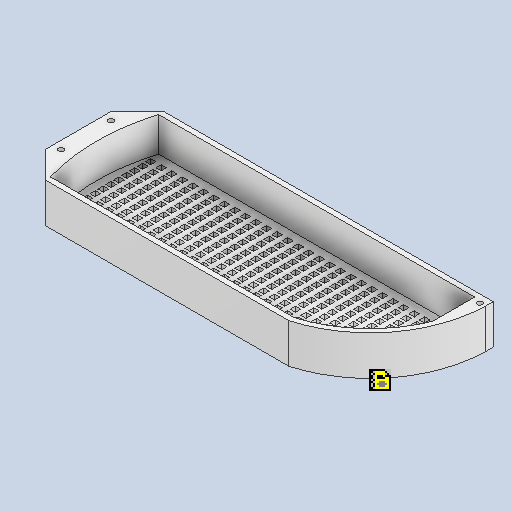
# Autodesk Inventor part: Box
Saved by Autodesk Inventor 2024 (Build 280153000, 153)
## iProperties
Created: 2023-11-02
Part Number: Box
Material: PVC, Unplasticized
Document SubType Name: Modeling
Designer: furqa
Density: 1.29 g/cm^3
Appearance: Smooth - White
Mass: 23.7695 g
Surface Area: 226.35 cm^2
Volume: 18.426 cm^3
Author: furqa
Autodesk Inventor part; units mm, degrees
(part 1 of 2)
ref_plane "YZ Plane" through (0, 0, 0) normal (1, 0, 0) x (0, 1, 0)
ref_plane "XZ Plane" through (0, 0, 0) normal (0, 1, 0) x (-1, 0, 0)
ref_plane "XY Plane" through (0, 0, 0) normal (0, 0, 1) x (1, 0, 0)
sketch "Sketch2" plane through (0, 0, 0) normal (0, 1, 0) x (-1, 0, 0)
  line L0 (0, 0) -> (125, 0)
  line L1 (125, 45) -> (0, 45)
  line L2 (0, 45) -> (0, 0)
  line L3 (125, 45) -> (135, 35)
  line L4 (125, 45) -> (139.1421, 45) construction
  line L5 (125, 0) -> (135, 10)
  line L6 (125, 0) -> (139.1421, 0) construction
  line L7 (135, 35) -> (135, 10)
  dimension "d3" = 45
  dimension "d4" = 45
  constraints: 16 end point, 3 horizontal, 2 equal length, 1 parallel
  measures "d3" angle of L3 L4
  measures "d4" angle of L6 L5
extrude "Extrusion2" add sketch "Sketch2" along normal blind 15
sketch "Sketch3" plane through (-135, 0, 10) normal (-0.7071, 0, -0.7071) x (-0.7071, 0, 0.7071)
  point P0 (-102.5305, 0)
sketch "Sketch4" plane through (0, 15, 0) normal (0, 1, 0) x (1, 0, 0)
  line L0 (-32.5163, -43) -> (-125, -43)
  line L1 (-125, -2) -> (-2, -2)
  line L2 (-2, -2) -> (-2, -4.6897)
  line L3 (0, -45) -> (0, 0) projected
  line L4 (0, 0) -> (-125, 0) projected
  line L5 (-125, -45) -> (0, -45) projected
  line L6 (-135, -10) -> (-135, -35) projected
  arc A0 (-32.5163, -45) -> (0, -1) centre (-44.7799, -1.9222) ccw
  arc A1 (-32.5163, -43) -> (-2, -4.6897) centre (-44.7799, -1.9222) ccw
  arc A2 (-125, -2) -> (-125, -43) centre (-56.4583, -22.5) ccw
  line L7 (-125, -45) -> (-125, -43)
  line L8 (-125, -2) -> (-125, 0)
  line L9 (-182.7929, -3.5) -> (-184.7929, -3.5)
  line L10 (-184.7929, -3.5) -> (-184.7929, -5.5)
  line L11 (-184.7929, -5.5) -> (-182.7929, -5.5)
  line L12 (-182.7929, -5.5) -> (-182.7929, -3.5)
  line L13 (0, 0) -> (-125, 0)
  line L14 (-125, 0) -> (-135, -10) projected
  line L15 (-135, -10) -> (-135, -35)
  line L16 (-135, -35) -> (-125, -45) projected
  line L17 (-125, -45) -> (-32.5163, -45)
  arc A3 (-32.5163, -45) -> (0, 0) centre (-44.9131, -1.7944) ccw
  point P0 (-135, -22.5)
  point P1 (-125, -22.5)
  point P2 (0, -2.8444)
  point P3 (-125, -22.5)
  point P4 (-128, -22.5)
  dimension "d11" = 2
  dimension "d12" = 2
  dimension "d34" = 2
  dimension "d62" = 2
  dimension "d63" = 2
  dimension "d64" = 1.5
  constraints: 24 end point, 9 point on circle, 5 parallel, 4 centre point, 2 horizontal, 2 point on line, 2 vertical, 1 coincident, 1 collinear, 1 midpoint, 1 perpendicular
  measures "d11" distance between parallel lines of L3 L2
  measures "d12" distance between parallel lines of L4 L1
  measures "d34" distance between parallel lines of L5 L0
  measures "d62" distance of L9.start L9.end
  measures "d63" distance of L11.end L9.start
  measures "d64" distance between parallel lines of L1 L9
extrude "Extrusion3" cut sketch "Sketch4" against normal blind 15 contours A0 A3 L3 L5
extrude "Extrusion4" cut sketch "Sketch4" against normal blind 13 contours L0 A2 L1 L2 A1
sketch "Sketch11" plane through (0, 2, 0) normal (0, 1, 0) x (1, 0, 0)
  point P0 (0, 0)
sketch "Sketch12" plane through (0, 2, 0) normal (0, 1, 0) x (1, 0, 0)
  line L0 (-125, -5) -> (-123, -5)
  line L1 (-123, -5) -> (-123, -7)
  line L2 (-123, -7) -> (-125, -7)
  line L3 (-125, -7) -> (-125, -5)
  line L4 (-125, -2) -> (-2, -2) projected
  arc A0 (-125, -2) -> (-125, -43) centre (-56.4583, -22.5) ccw projected
  line L5 (-121, -5) -> (-119, -5)
  line L6 (-119, -5) -> (-119, -7)
  line L7 (-119, -7) -> (-121, -7)
  line L8 (-121, -7) -> (-121, -5)
  line L9 (-117, -5) -> (-115, -5)
  line L10 (-115, -5) -> (-115, -7)
  line L11 (-115, -7) -> (-117, -7)
  line L12 (-117, -7) -> (-117, -5)
  line L13 (-113, -5) -> (-111, -5)
  line L14 (-111, -5) -> (-111, -7)
  line L15 (-111, -7) -> (-113, -7)
  line L16 (-113, -7) -> (-113, -5)
  line L17 (-109, -5) -> (-107, -5)
  line L18 (-107, -5) -> (-107, -7)
  line L19 (-107, -7) -> (-109, -7)
  line L20 (-109, -7) -> (-109, -5)
  line L21 (-105, -5) -> (-103, -5)
  line L22 (-103, -5) -> (-103, -7)
  line L23 (-103, -7) -> (-105, -7)
  line L24 (-105, -7) -> (-105, -5)
  line L25 (-101, -5) -> (-99, -5)
  line L26 (-99, -5) -> (-99, -7)
  line L27 (-99, -7) -> (-101, -7)
  line L28 (-101, -7) -> (-101, -5)
  line L29 (-97, -5) -> (-95, -5)
  line L30 (-95, -5) -> (-95, -7)
  line L31 (-95, -7) -> (-97, -7)
  line L32 (-97, -7) -> (-97, -5)
  line L33 (-93, -5) -> (-91, -5)
  line L34 (-91, -5) -> (-91, -7)
  line L35 (-91, -7) -> (-93, -7)
  line L36 (-93, -7) -> (-93, -5)
  line L37 (-89, -5) -> (-87, -5)
  line L38 (-87, -5) -> (-87, -7)
  line L39 (-87, -7) -> (-89, -7)
  line L40 (-89, -7) -> (-89, -5)
  line L41 (-85, -5) -> (-83, -5)
  line L42 (-83, -5) -> (-83, -7)
  line L43 (-83, -7) -> (-85, -7)
  line L44 (-85, -7) -> (-85, -5)
  line L45 (-81, -5) -> (-79, -5)
  line L46 (-79, -5) -> (-79, -7)
  line L47 (-79, -7) -> (-81, -7)
  line L48 (-81, -7) -> (-81, -5)
  line L49 (-77, -5) -> (-75, -5)
  line L50 (-75, -5) -> (-75, -7)
  line L51 (-75, -7) -> (-77, -7)
  line L52 (-77, -7) -> (-77, -5)
  line L53 (-73, -5) -> (-71, -5)
  line L54 (-71, -5) -> (-71, -7)
  line L55 (-71, -7) -> (-73, -7)
  line L56 (-73, -7) -> (-73, -5)
  line L57 (-69, -5) -> (-67, -5)
  line L58 (-67, -5) -> (-67, -7)
  line L59 (-67, -7) -> (-69, -7)
  line L60 (-69, -7) -> (-69, -5)
  line L61 (-65, -5) -> (-63, -5)
  line L62 (-63, -5) -> (-63, -7)
  line L63 (-63, -7) -> (-65, -7)
  line L64 (-65, -7) -> (-65, -5)
  line L65 (-61, -5) -> (-59, -5)
  line L66 (-59, -5) -> (-59, -7)
  line L67 (-59, -7) -> (-61, -7)
  line L68 (-61, -7) -> (-61, -5)
  line L69 (-57, -5) -> (-55, -5)
  line L70 (-55, -5) -> (-55, -7)
  line L71 (-55, -7) -> (-57, -7)
  line L72 (-57, -7) -> (-57, -5)
  line L73 (-53, -5) -> (-51, -5)
  line L74 (-51, -5) -> (-51, -7)
  line L75 (-51, -7) -> (-53, -7)
  line L76 (-53, -7) -> (-53, -5)
  line L77 (-49, -5) -> (-47, -5)
  line L78 (-47, -5) -> (-47, -7)
  line L79 (-47, -7) -> (-49, -7)
  line L80 (-49, -7) -> (-49, -5)
  line L81 (-45, -5) -> (-43, -5)
  line L82 (-43, -5) -> (-43, -7)
  line L83 (-43, -7) -> (-45, -7)
  line L84 (-45, -7) -> (-45, -5)
  line L85 (-41, -5) -> (-39, -5)
  line L86 (-39, -5) -> (-39, -7)
  line L87 (-39, -7) -> (-41, -7)
  line L88 (-41, -7) -> (-41, -5)
  line L89 (-37, -5) -> (-35, -5)
  line L90 (-35, -5) -> (-35, -7)
  line L91 (-35, -7) -> (-37, -7)
  line L92 (-37, -7) -> (-37, -5)
  line L93 (-33, -5) -> (-31, -5)
  line L94 (-31, -5) -> (-31, -7)
  line L95 (-31, -7) -> (-33, -7)
  line L96 (-33, -7) -> (-33, -5)
  line L97 (-125, -8) -> (-123, -8)
  line L98 (-123, -8) -> (-123, -10)
  line L99 (-123, -10) -> (-125, -10)
  line L100 (-125, -10) -> (-125, -8)
  line L101 (-121, -8) -> (-119, -8)
  line L102 (-119, -8) -> (-119, -10)
  line L103 (-119, -10) -> (-121, -10)
  line L104 (-121, -10) -> (-121, -8)
  line L105 (-117, -8) -> (-115, -8)
  line L106 (-115, -8) -> (-115, -10)
  line L107 (-115, -10) -> (-117, -10)
  line L108 (-117, -10) -> (-117, -8)
  line L109 (-113, -8) -> (-111, -8)
  line L110 (-111, -8) -> (-111, -10)
  line L111 (-111, -10) -> (-113, -10)
  line L112 (-113, -10) -> (-113, -8)
  line L113 (-109, -8) -> (-107, -8)
  line L114 (-107, -8) -> (-107, -10)
  line L115 (-107, -10) -> (-109, -10)
  line L116 (-109, -10) -> (-109, -8)
  line L117 (-105, -8) -> (-103, -8)
  line L118 (-103, -8) -> (-103, -10)
  line L119 (-103, -10) -> (-105, -10)
  line L120 (-105, -10) -> (-105, -8)
  line L121 (-101, -8) -> (-99, -8)
  line L122 (-99, -8) -> (-99, -10)
  line L123 (-99, -10) -> (-101, -10)
  line L124 (-101, -10) -> (-101, -8)
  line L125 (-97, -8) -> (-95, -8)
  line L126 (-95, -8) -> (-95, -10)
  line L127 (-95, -10) -> (-97, -10)
  line L128 (-97, -10) -> (-97, -8)
  line L129 (-93, -8) -> (-91, -8)
  line L130 (-91, -8) -> (-91, -10)
  line L131 (-91, -10) -> (-93, -10)
  line L132 (-93, -10) -> (-93, -8)
  line L133 (-89, -8) -> (-87, -8)
  line L134 (-87, -8) -> (-87, -10)
  line L135 (-87, -10) -> (-89, -10)
  line L136 (-89, -10) -> (-89, -8)
  line L137 (-85, -8) -> (-83, -8)
  line L138 (-83, -8) -> (-83, -10)
  line L139 (-83, -10) -> (-85, -10)
  line L140 (-85, -10) -> (-85, -8)
  line L141 (-81, -8) -> (-79, -8)
  line L142 (-79, -8) -> (-79, -10)
  line L143 (-79, -10) -> (-81, -10)
  line L144 (-81, -10) -> (-81, -8)
  line L145 (-77, -8) -> (-75, -8)
  line L146 (-75, -8) -> (-75, -10)
  line L147 (-75, -10) -> (-77, -10)
  line L148 (-77, -10) -> (-77, -8)
  line L149 (-73, -8) -> (-71, -8)
  line L150 (-71, -8) -> (-71, -10)
  line L151 (-71, -10) -> (-73, -10)
  line L152 (-73, -10) -> (-73, -8)
  line L153 (-69, -8) -> (-67, -8)
  line L154 (-67, -8) -> (-67, -10)
  line L155 (-67, -10) -> (-69, -10)
  line L156 (-69, -10) -> (-69, -8)
  line L157 (-65, -8) -> (-63, -8)
  line L158 (-63, -8) -> (-63, -10)
  line L159 (-63, -10) -> (-65, -10)
  line L160 (-65, -10) -> (-65, -8)
  line L161 (-61, -8) -> (-59, -8)
  line L162 (-59, -8) -> (-59, -10)
  line L163 (-59, -10) -> (-61, -10)
  line L164 (-61, -10) -> (-61, -8)
  line L165 (-57, -8) -> (-55, -8)
  line L166 (-55, -8) -> (-55, -10)
  line L167 (-55, -10) -> (-57, -10)
  line L168 (-57, -10) -> (-57, -8)
  line L169 (-53, -8) -> (-51, -8)
  line L170 (-51, -8) -> (-51, -10)
  line L171 (-51, -10) -> (-53, -10)
  line L172 (-53, -10) -> (-53, -8)
  line L173 (-49, -8) -> (-47, -8)
  line L174 (-47, -8) -> (-47, -10)
  line L175 (-47, -10) -> (-49, -10)
  line L176 (-49, -10) -> (-49, -8)
  line L177 (-45, -8) -> (-43, -8)
  line L178 (-43, -8) -> (-43, -10)
  line L179 (-43, -10) -> (-45, -10)
  line L180 (-45, -10) -> (-45, -8)
  line L181 (-41, -8) -> (-39, -8)
  line L182 (-39, -8) -> (-39, -10)
  line L183 (-39, -10) -> (-41, -10)
  line L184 (-41, -10) -> (-41, -8)
  line L185 (-37, -8) -> (-35, -8)
  line L186 (-35, -8) -> (-35, -10)
  line L187 (-35, -10) -> (-37, -10)
  line L188 (-37, -10) -> (-37, -8)
  line L189 (-33, -8) -> (-31, -8)
  line L190 (-31, -8) -> (-31, -10)
  line L191 (-31, -10) -> (-33, -10)
  line L192 (-33, -10) -> (-33, -8)
  line L193 (-125, -11) -> (-123, -11)
  line L194 (-123, -11) -> (-123, -13)
  line L195 (-123, -13) -> (-125, -13)
  line L196 (-125, -13) -> (-125, -11)
  line L197 (-121, -11) -> (-119, -11)
  line L198 (-119, -11) -> (-119, -13)
  line L199 (-119, -13) -> (-121, -13)
  line L200 (-121, -13) -> (-121, -11)
  line L201 (-117, -11) -> (-115, -11)
  line L202 (-115, -11) -> (-115, -13)
  line L203 (-115, -13) -> (-117, -13)
  line L204 (-117, -13) -> (-117, -11)
  line L205 (-113, -11) -> (-111, -11)
  line L206 (-111, -11) -> (-111, -13)
  line L207 (-111, -13) -> (-113, -13)
  line L208 (-113, -13) -> (-113, -11)
  line L209 (-109, -11) -> (-107, -11)
  line L210 (-107, -11) -> (-107, -13)
  line L211 (-107, -13) -> (-109, -13)
  line L212 (-109, -13) -> (-109, -11)
  line L213 (-105, -11) -> (-103, -11)
  line L214 (-103, -11) -> (-103, -13)
  line L215 (-103, -13) -> (-105, -13)
  line L216 (-105, -13) -> (-105, -11)
  line L217 (-101, -11) -> (-99, -11)
  line L218 (-99, -11) -> (-99, -13)
  line L219 (-99, -13) -> (-101, -13)
  line L220 (-101, -13) -> (-101, -11)
  line L221 (-97, -11) -> (-95, -11)
  line L222 (-95, -11) -> (-95, -13)
  line L223 (-95, -13) -> (-97, -13)
  line L224 (-97, -13) -> (-97, -11)
  line L225 (-93, -11) -> (-91, -11)
  line L226 (-91, -11) -> (-91, -13)
  line L227 (-91, -13) -> (-93, -13)
  line L228 (-93, -13) -> (-93, -11)
  line L229 (-89, -11) -> (-87, -11)
  line L230 (-87, -11) -> (-87, -13)
  line L231 (-87, -13) -> (-89, -13)
  line L232 (-89, -13) -> (-89, -11)
  line L233 (-85, -11) -> (-83, -11)
  line L234 (-83, -11) -> (-83, -13)
  line L235 (-83, -13) -> (-85, -13)
  line L236 (-85, -13) -> (-85, -11)
  line L237 (-81, -11) -> (-79, -11)
  line L238 (-79, -11) -> (-79, -13)
  line L239 (-79, -13) -> (-81, -13)
  line L240 (-81, -13) -> (-81, -11)
  line L241 (-77, -11) -> (-75, -11)
  line L242 (-75, -11) -> (-75, -13)
  line L243 (-75, -13) -> (-77, -13)
  line L244 (-77, -13) -> (-77, -11)
  line L245 (-73, -11) -> (-71, -11)
  line L246 (-71, -11) -> (-71, -13)
  line L247 (-71, -13) -> (-73, -13)
  line L248 (-73, -13) -> (-73, -11)
  line L249 (-69, -11) -> (-67, -11)
  line L250 (-67, -11) -> (-67, -13)
  line L251 (-67, -13) -> (-69, -13)
  line L252 (-69, -13) -> (-69, -11)
  line L253 (-65, -11) -> (-63, -11)
  line L254 (-63, -11) -> (-63, -13)
  line L255 (-63, -13) -> (-65, -13)
  line L256 (-65, -13) -> (-65, -11)
  line L257 (-61, -11) -> (-59, -11)
  line L258 (-59, -11) -> (-59, -13)
  line L259 (-59, -13) -> (-61, -13)
  line L260 (-61, -13) -> (-61, -11)
  line L261 (-57, -11) -> (-55, -11)
  line L262 (-55, -11) -> (-55, -13)
  line L263 (-55, -13) -> (-57, -13)
  line L264 (-57, -13) -> (-57, -11)
  line L265 (-53, -11) -> (-51, -11)
  line L266 (-51, -11) -> (-51, -13)
  line L267 (-51, -13) -> (-53, -13)
  line L268 (-53, -13) -> (-53, -11)
  line L269 (-49, -11) -> (-47, -11)
  line L270 (-47, -11) -> (-47, -13)
  line L271 (-47, -13) -> (-49, -13)
  line L272 (-49, -13) -> (-49, -11)
  line L273 (-45, -11) -> (-43, -11)
  line L274 (-43, -11) -> (-43, -13)
  line L275 (-43, -13) -> (-45, -13)
  line L276 (-45, -13) -> (-45, -11)
  line L277 (-41, -11) -> (-39, -11)
  line L278 (-39, -11) -> (-39, -13)
  line L279 (-39, -13) -> (-41, -13)
  line L280 (-41, -13) -> (-41, -11)
  line L281 (-37, -11) -> (-35, -11)
  line L282 (-35, -11) -> (-35, -13)
  line L283 (-35, -13) -> (-37, -13)
  line L284 (-37, -13) -> (-37, -11)
  line L285 (-33, -11) -> (-31, -11)
  line L286 (-31, -11) -> (-31, -13)
  line L287 (-31, -13) -> (-33, -13)
  line L288 (-33, -13) -> (-33, -11)
  line L289 (-125, -14) -> (-123, -14)
  line L290 (-123, -14) -> (-123, -16)
  line L291 (-123, -16) -> (-125, -16)
  line L292 (-125, -16) -> (-125, -14)
  line L293 (-121, -14) -> (-119, -14)
  line L294 (-119, -14) -> (-119, -16)
  line L295 (-119, -16) -> (-121, -16)
  line L296 (-121, -16) -> (-121, -14)
  line L297 (-117, -14) -> (-115, -14)
  line L298 (-115, -14) -> (-115, -16)
  line L299 (-115, -16) -> (-117, -16)
  line L300 (-117, -16) -> (-117, -14)
  line L301 (-113, -14) -> (-111, -14)
  line L302 (-111, -14) -> (-111, -16)
  line L303 (-111, -16) -> (-113, -16)
  line L304 (-113, -16) -> (-113, -14)
  line L305 (-109, -14) -> (-107, -14)
  line L306 (-107, -14) -> (-107, -16)
  line L307 (-107, -16) -> (-109, -16)
  line L308 (-109, -16) -> (-109, -14)
  line L309 (-105, -14) -> (-103, -14)
  line L310 (-103, -14) -> (-103, -16)
  line L311 (-103, -16) -> (-105, -16)
  line L312 (-105, -16) -> (-105, -14)
  line L313 (-101, -14) -> (-99, -14)
  line L314 (-99, -14) -> (-99, -16)
  line L315 (-99, -16) -> (-101, -16)
  line L316 (-101, -16) -> (-101, -14)
  line L317 (-97, -14) -> (-95, -14)
  line L318 (-95, -14) -> (-95, -16)
  line L319 (-95, -16) -> (-97, -16)
  line L320 (-97, -16) -> (-97, -14)
  line L321 (-93, -14) -> (-91, -14)
  line L322 (-91, -14) -> (-91, -16)
  line L323 (-91, -16) -> (-93, -16)
  line L324 (-93, -16) -> (-93, -14)
  line L325 (-89, -14) -> (-87, -14)
  line L326 (-87, -14) -> (-87, -16)
  line L327 (-87, -16) -> (-89, -16)
  line L328 (-89, -16) -> (-89, -14)
  line L329 (-85, -14) -> (-83, -14)
  line L330 (-83, -14) -> (-83, -16)
  line L331 (-83, -16) -> (-85, -16)
  line L332 (-85, -16) -> (-85, -14)
  line L333 (-81, -14) -> (-79, -14)
  line L334 (-79, -14) -> (-79, -16)
  line L335 (-79, -16) -> (-81, -16)
  line L336 (-81, -16) -> (-81, -14)
  line L337 (-77, -14) -> (-75, -14)
  line L338 (-75, -14) -> (-75, -16)
  line L339 (-75, -16) -> (-77, -16)
  line L340 (-77, -16) -> (-77, -14)
  line L341 (-73, -14) -> (-71, -14)
  line L342 (-71, -14) -> (-71, -16)
  line L343 (-71, -16) -> (-73, -16)
  line L344 (-73, -16) -> (-73, -14)
  line L345 (-69, -14) -> (-67, -14)
  line L346 (-67, -14) -> (-67, -16)
  line L347 (-67, -16) -> (-69, -16)
  line L348 (-69, -16) -> (-69, -14)
  line L349 (-65, -14) -> (-63, -14)
  line L350 (-63, -14) -> (-63, -16)
  line L351 (-63, -16) -> (-65, -16)
  line L352 (-65, -16) -> (-65, -14)
  line L353 (-61, -14) -> (-59, -14)
  line L354 (-59, -14) -> (-59, -16)
  line L355 (-59, -16) -> (-61, -16)
  line L356 (-61, -16) -> (-61, -14)
  line L357 (-57, -14) -> (-55, -14)
  line L358 (-55, -14) -> (-55, -16)
  line L359 (-55, -16) -> (-57, -16)
  line L360 (-57, -16) -> (-57, -14)
  line L361 (-53, -14) -> (-51, -14)
  line L362 (-51, -14) -> (-51, -16)
  line L363 (-51, -16) -> (-53, -16)
  line L364 (-53, -16) -> (-53, -14)
  line L365 (-49, -14) -> (-47, -14)
  line L366 (-47, -14) -> (-47, -16)
  line L367 (-47, -16) -> (-49, -16)
  line L368 (-49, -16) -> (-49, -14)
  line L369 (-45, -14) -> (-43, -14)
  line L370 (-43, -14) -> (-43, -16)
  line L371 (-43, -16) -> (-45, -16)
  line L372 (-45, -16) -> (-45, -14)
  line L373 (-41, -14) -> (-39, -14)
  line L374 (-39, -14) -> (-39, -16)
  line L375 (-39, -16) -> (-41, -16)
  line L376 (-41, -16) -> (-41, -14)
  line L377 (-37, -14) -> (-35, -14)
  line L378 (-35, -14) -> (-35, -16)
  line L379 (-35, -16) -> (-37, -16)
  line L380 (-37, -16) -> (-37, -14)
  line L381 (-33, -14) -> (-31, -14)
  line L382 (-31, -14) -> (-31, -16)
  line L383 (-31, -16) -> (-33, -16)
  line L384 (-33, -16) -> (-33, -14)
  line L385 (-125, -17) -> (-123, -17)
  line L386 (-123, -17) -> (-123, -19)
  line L387 (-123, -19) -> (-125, -19)
  line L388 (-125, -19) -> (-125, -17)
  line L389 (-121, -17) -> (-119, -17)
  line L390 (-119, -17) -> (-119, -19)
  line L391 (-119, -19) -> (-121, -19)
  line L392 (-121, -19) -> (-121, -17)
  line L393 (-117, -17) -> (-115, -17)
  line L394 (-115, -17) -> (-115, -19)
  line L395 (-115, -19) -> (-117, -19)
  line L396 (-117, -19) -> (-117, -17)
  line L397 (-113, -17) -> (-111, -17)
  line L398 (-111, -17) -> (-111, -19)
  line L399 (-111, -19) -> (-113, -19)
  line L400 (-113, -19) -> (-113, -17)
  line L401 (-109, -17) -> (-107, -17)
  line L402 (-107, -17) -> (-107, -19)
  line L403 (-107, -19) -> (-109, -19)
  line L404 (-109, -19) -> (-109, -17)
  line L405 (-105, -17) -> (-103, -17)
  line L406 (-103, -17) -> (-103, -19)
  line L407 (-103, -19) -> (-105, -19)
  line L408 (-105, -19) -> (-105, -17)
  line L409 (-101, -17) -> (-99, -17)
  line L410 (-99, -17) -> (-99, -19)
  line L411 (-99, -19) -> (-101, -19)
  line L412 (-101, -19) -> (-101, -17)
  line L413 (-97, -17) -> (-95, -17)
  line L414 (-95, -17) -> (-95, -19)
  line L415 (-95, -19) -> (-97, -19)
  line L416 (-97, -19) -> (-97, -17)
  line L417 (-93, -17) -> (-91, -17)
  line L418 (-91, -17) -> (-91, -19)
  line L419 (-91, -19) -> (-93, -19)
  line L420 (-93, -19) -> (-93, -17)
  line L421 (-89, -17) -> (-87, -17)
  line L422 (-87, -17) -> (-87, -19)
  line L423 (-87, -19) -> (-89, -19)
  line L424 (-89, -19) -> (-89, -17)
  line L425 (-85, -17) -> (-83, -17)
  line L426 (-83, -17) -> (-83, -19)
  line L427 (-83, -19) -> (-85, -19)
  line L428 (-85, -19) -> (-85, -17)
  line L429 (-81, -17) -> (-79, -17)
  line L430 (-79, -17) -> (-79, -19)
  line L431 (-79, -19) -> (-81, -19)
  line L432 (-81, -19) -> (-81, -17)
  line L433 (-77, -17) -> (-75, -17)
  line L434 (-75, -17) -> (-75, -19)
  line L435 (-75, -19) -> (-77, -19)
  line L436 (-77, -19) -> (-77, -17)
  line L437 (-73, -17) -> (-71, -17)
  line L438 (-71, -17) -> (-71, -19)
  line L439 (-71, -19) -> (-73, -19)
  line L440 (-73, -19) -> (-73, -17)
  line L441 (-69, -17) -> (-67, -17)
  line L442 (-67, -17) -> (-67, -19)
  line L443 (-67, -19) -> (-69, -19)
  line L444 (-69, -19) -> (-69, -17)
  line L445 (-65, -17) -> (-63, -17)
  line L446 (-63, -17) -> (-63, -19)
  line L447 (-63, -19) -> (-65, -19)
  line L448 (-65, -19) -> (-65, -17)
  line L449 (-61, -17) -> (-59, -17)
  line L450 (-59, -17) -> (-59, -19)
  line L451 (-59, -19) -> (-61, -19)
  line L452 (-61, -19) -> (-61, -17)
  line L453 (-57, -17) -> (-55, -17)
  line L454 (-55, -17) -> (-55, -19)
  line L455 (-55, -19) -> (-57, -19)
  line L456 (-57, -19) -> (-57, -17)
  line L457 (-53, -17) -> (-51, -17)
  line L458 (-51, -17) -> (-51, -19)
  line L459 (-51, -19) -> (-53, -19)
  line L460 (-53, -19) -> (-53, -17)
  line L461 (-49, -17) -> (-47, -17)
  line L462 (-47, -17) -> (-47, -19)
  line L463 (-47, -19) -> (-49, -19)
  line L464 (-49, -19) -> (-49, -17)
  line L465 (-45, -17) -> (-43, -17)
  line L466 (-43, -17) -> (-43, -19)
  line L467 (-43, -19) -> (-45, -19)
  line L468 (-45, -19) -> (-45, -17)
  line L469 (-41, -17) -> (-39, -17)
  line L470 (-39, -17) -> (-39, -19)
  line L471 (-39, -19) -> (-41, -19)
  line L472 (-41, -19) -> (-41, -17)
  line L473 (-37, -17) -> (-35, -17)
  line L474 (-35, -17) -> (-35, -19)
  line L475 (-35, -19) -> (-37, -19)
  line L476 (-37, -19) -> (-37, -17)
  line L477 (-33, -17) -> (-31, -17)
  line L478 (-31, -17) -> (-31, -19)
  line L479 (-31, -19) -> (-33, -19)
  line L480 (-33, -19) -> (-33, -17)
  line L481 (-125, -20) -> (-123, -20)
  line L482 (-123, -20) -> (-123, -22)
  line L483 (-123, -22) -> (-125, -22)
  line L484 (-125, -22) -> (-125, -20)
  line L485 (-121, -20) -> (-119, -20)
  line L486 (-119, -20) -> (-119, -22)
  line L487 (-119, -22) -> (-121, -22)
  line L488 (-121, -22) -> (-121, -20)
  line L489 (-117, -20) -> (-115, -20)
  line L490 (-115, -20) -> (-115, -22)
  line L491 (-115, -22) -> (-117, -22)
  line L492 (-117, -22) -> (-117, -20)
  line L493 (-113, -20) -> (-111, -20)
  line L494 (-111, -20) -> (-111, -22)
  line L495 (-111, -22) -> (-113, -22)
  line L496 (-113, -22) -> (-113, -20)
  line L497 (-109, -20) -> (-107, -20)
  line L498 (-107, -20) -> (-107, -22)
  line L499 (-107, -22) -> (-109, -22)
  line L500 (-109, -22) -> (-109, -20)
  line L501 (-105, -20) -> (-103, -20)
  line L502 (-103, -20) -> (-103, -22)
  line L503 (-103, -22) -> (-105, -22)
  line L504 (-105, -22) -> (-105, -20)
  line L505 (-101, -20) -> (-99, -20)
  line L506 (-99, -20) -> (-99, -22)
  line L507 (-99, -22) -> (-101, -22)
  line L508 (-101, -22) -> (-101, -20)
  line L509 (-97, -20) -> (-95, -20)
  line L510 (-95, -20) -> (-95, -22)
  line L511 (-95, -22) -> (-97, -22)
  line L512 (-97, -22) -> (-97, -20)
  line L513 (-93, -20) -> (-91, -20)
  line L514 (-91, -20) -> (-91, -22)
  line L515 (-91, -22) -> (-93, -22)
  line L516 (-93, -22) -> (-93, -20)
  line L517 (-89, -20) -> (-87, -20)
  line L518 (-87, -20) -> (-87, -22)
  line L519 (-87, -22) -> (-89, -22)
  line L520 (-89, -22) -> (-89, -20)
  line L521 (-85, -20) -> (-83, -20)
  line L522 (-83, -20) -> (-83, -22)
  line L523 (-83, -22) -> (-85, -22)
  line L524 (-85, -22) -> (-85, -20)
  line L525 (-81, -20) -> (-79, -20)
  line L526 (-79, -20) -> (-79, -22)
  line L527 (-79, -22) -> (-81, -22)
  line L528 (-81, -22) -> (-81, -20)
  line L529 (-77, -20) -> (-75, -20)
  line L530 (-75, -20) -> (-75, -22)
  line L531 (-75, -22) -> (-77, -22)
  line L532 (-77, -22) -> (-77, -20)
  line L533 (-73, -20) -> (-71, -20)
  line L534 (-71, -20) -> (-71, -22)
  line L535 (-71, -22) -> (-73, -22)
  line L536 (-73, -22) -> (-73, -20)
  line L537 (-69, -20) -> (-67, -20)
  line L538 (-67, -20) -> (-67, -22)
  line L539 (-67, -22) -> (-69, -22)
  line L540 (-69, -22) -> (-69, -20)
  line L541 (-65, -20) -> (-63, -20)
  line L542 (-63, -20) -> (-63, -22)
  line L543 (-63, -22) -> (-65, -22)
  line L544 (-65, -22) -> (-65, -20)
  line L545 (-61, -20) -> (-59, -20)
  line L546 (-59, -20) -> (-59, -22)
  line L547 (-59, -22) -> (-61, -22)
  line L548 (-61, -22) -> (-61, -20)
  line L549 (-57, -20) -> (-55, -20)
  line L550 (-55, -20) -> (-55, -22)
  line L551 (-55, -22) -> (-57, -22)
  line L552 (-57, -22) -> (-57, -20)
  line L553 (-53, -20) -> (-51, -20)
  line L554 (-51, -20) -> (-51, -22)
  line L555 (-51, -22) -> (-53, -22)
  line L556 (-53, -22) -> (-53, -20)
  line L557 (-49, -20) -> (-47, -20)
  line L558 (-47, -20) -> (-47, -22)
  line L559 (-47, -22) -> (-49, -22)
  line L560 (-49, -22) -> (-49, -20)
  line L561 (-45, -20) -> (-43, -20)
  line L562 (-43, -20) -> (-43, -22)
  line L563 (-43, -22) -> (-45, -22)
  line L564 (-45, -22) -> (-45, -20)
  line L565 (-41, -20) -> (-39, -20)
  line L566 (-39, -20) -> (-39, -22)
  line L567 (-39, -22) -> (-41, -22)
  line L568 (-41, -22) -> (-41, -20)
  line L569 (-37, -20) -> (-35, -20)
  line L570 (-35, -20) -> (-35, -22)
  line L571 (-35, -22) -> (-37, -22)
  line L572 (-37, -22) -> (-37, -20)
  line L573 (-33, -20) -> (-31, -20)
  line L574 (-31, -20) -> (-31, -22)
  line L575 (-31, -22) -> (-33, -22)
  line L576 (-33, -22) -> (-33, -20)
  line L577 (-125, -23) -> (-123, -23)
  line L578 (-123, -23) -> (-123, -25)
  line L579 (-123, -25) -> (-125, -25)
  line L580 (-125, -25) -> (-125, -23)
  line L581 (-121, -23) -> (-119, -23)
  line L582 (-119, -23) -> (-119, -25)
  line L583 (-119, -25) -> (-121, -25)
  line L584 (-121, -25) -> (-121, -23)
  line L585 (-117, -23) -> (-115, -23)
  line L586 (-115, -23) -> (-115, -25)
  line L587 (-115, -25) -> (-117, -25)
  line L588 (-117, -25) -> (-117, -23)
  line L589 (-113, -23) -> (-111, -23)
  line L590 (-111, -23) -> (-111, -25)
  line L591 (-111, -25) -> (-113, -25)
  line L592 (-113, -25) -> (-113, -23)
  line L593 (-109, -23) -> (-107, -23)
  line L594 (-107, -23) -> (-107, -25)
  line L595 (-107, -25) -> (-109, -25)
  line L596 (-109, -25) -> (-109, -23)
  line L597 (-105, -23) -> (-103, -23)
  line L598 (-103, -23) -> (-103, -25)
  line L599 (-103, -25) -> (-105, -25)
  line L600 (-105, -25) -> (-105, -23)
  line L601 (-101, -23) -> (-99, -23)
  line L602 (-99, -23) -> (-99, -25)
  line L603 (-99, -25) -> (-101, -25)
  line L604 (-101, -25) -> (-101, -23)
  line L605 (-97, -23) -> (-95, -23)
  line L606 (-95, -23) -> (-95, -25)
  line L607 (-95, -25) -> (-97, -25)
  line L608 (-97, -25) -> (-97, -23)
  line L609 (-93, -23) -> (-91, -23)
  line L610 (-91, -23) -> (-91, -25)
  line L611 (-91, -25) -> (-93, -25)
  line L612 (-93, -25) -> (-93, -23)
  line L613 (-89, -23) -> (-87, -23)
  line L614 (-87, -23) -> (-87, -25)
  line L615 (-87, -25) -> (-89, -25)
  line L616 (-89, -25) -> (-89, -23)
  line L617 (-85, -23) -> (-83, -23)
  line L618 (-83, -23) -> (-83, -25)
  line L619 (-83, -25) -> (-85, -25)
  line L620 (-85, -25) -> (-85, -23)
  line L621 (-81, -23) -> (-79, -23)
  line L622 (-79, -23) -> (-79, -25)
  line L623 (-79, -25) -> (-81, -25)
  line L624 (-81, -25) -> (-81, -23)
  line L625 (-77, -23) -> (-75, -23)
  line L626 (-75, -23) -> (-75, -25)
  line L627 (-75, -25) -> (-77, -25)
  line L628 (-77, -25) -> (-77, -23)
  line L629 (-73, -23) -> (-71, -23)
  line L630 (-71, -23) -> (-71, -25)
  line L631 (-71, -25) -> (-73, -25)
  line L632 (-73, -25) -> (-73, -23)
  line L633 (-69, -23) -> (-67, -23)
  line L634 (-67, -23) -> (-67, -25)
  line L635 (-67, -25) -> (-69, -25)
  line L636 (-69, -25) -> (-69, -23)
  line L637 (-65, -23) -> (-63, -23)
  line L638 (-63, -23) -> (-63, -25)
  line L639 (-63, -25) -> (-65, -25)
  line L640 (-65, -25) -> (-65, -23)
  line L641 (-61, -23) -> (-59, -23)
  line L642 (-59, -23) -> (-59, -25)
  line L643 (-59, -25) -> (-61, -25)
  line L644 (-61, -25) -> (-61, -23)
  line L645 (-57, -23) -> (-55, -23)
  line L646 (-55, -23) -> (-55, -25)
  line L647 (-55, -25) -> (-57, -25)
  line L648 (-57, -25) -> (-57, -23)
  line L649 (-53, -23) -> (-51, -23)
  line L650 (-51, -23) -> (-51, -25)
  line L651 (-51, -25) -> (-53, -25)
  line L652 (-53, -25) -> (-53, -23)
  line L653 (-49, -23) -> (-47, -23)
  line L654 (-47, -23) -> (-47, -25)
  line L655 (-47, -25) -> (-49, -25)
  line L656 (-49, -25) -> (-49, -23)
  line L657 (-45, -23) -> (-43, -23)
  line L658 (-43, -23) -> (-43, -25)
  line L659 (-43, -25) -> (-45, -25)
  line L660 (-45, -25) -> (-45, -23)
  line L661 (-41, -23) -> (-39, -23)
  line L662 (-39, -23) -> (-39, -25)
  line L663 (-39, -25) -> (-41, -25)
  line L664 (-41, -25) -> (-41, -23)
  line L665 (-37, -23) -> (-35, -23)
  line L666 (-35, -23) -> (-35, -25)
  line L667 (-35, -25) -> (-37, -25)
  line L668 (-37, -25) -> (-37, -23)
  line L669 (-33, -23) -> (-31, -23)
  line L670 (-31, -23) -> (-31, -25)
  line L671 (-31, -25) -> (-33, -25)
  line L672 (-33, -25) -> (-33, -23)
  line L673 (-125, -26) -> (-123, -26)
  line L674 (-123, -26) -> (-123, -28)
  line L675 (-123, -28) -> (-125, -28)
  line L676 (-125, -28) -> (-125, -26)
  line L677 (-121, -26) -> (-119, -26)
  line L678 (-119, -26) -> (-119, -28)
  line L679 (-119, -28) -> (-121, -28)
  line L680 (-121, -28) -> (-121, -26)
  line L681 (-117, -26) -> (-115, -26)
  line L682 (-115, -26) -> (-115, -28)
  line L683 (-115, -28) -> (-117, -28)
  line L684 (-117, -28) -> (-117, -26)
  line L685 (-113, -26) -> (-111, -26)
  line L686 (-111, -26) -> (-111, -28)
  line L687 (-111, -28) -> (-113, -28)
  line L688 (-113, -28) -> (-113, -26)
  line L689 (-109, -26) -> (-107, -26)
  line L690 (-107, -26) -> (-107, -28)
  line L691 (-107, -28) -> (-109, -28)
  line L692 (-109, -28) -> (-109, -26)
  line L693 (-105, -26) -> (-103, -26)
  line L694 (-103, -26) -> (-103, -28)
  line L695 (-103, -28) -> (-105, -28)
  line L696 (-105, -28) -> (-105, -26)
  line L697 (-101, -26) -> (-99, -26)
  line L698 (-99, -26) -> (-99, -28)
  line L699 (-99, -28) -> (-101, -28)
  line L700 (-101, -28) -> (-101, -26)
  line L701 (-97, -26) -> (-95, -26)
  line L702 (-95, -26) -> (-95, -28)
  line L703 (-95, -28) -> (-97, -28)
  line L704 (-97, -28) -> (-97, -26)
  line L705 (-93, -26) -> (-91, -26)
  line L706 (-91, -26) -> (-91, -28)
  line L707 (-91, -28) -> (-93, -28)
  line L708 (-93, -28) -> (-93, -26)
  line L709 (-89, -26) -> (-87, -26)
  line L710 (-87, -26) -> (-87, -28)
  line L711 (-87, -28) -> (-89, -28)
  line L712 (-89, -28) -> (-89, -26)
  line L713 (-85, -26) -> (-83, -26)
  line L714 (-83, -26) -> (-83, -28)
  line L715 (-83, -28) -> (-85, -28)
  line L716 (-85, -28) -> (-85, -26)
  line L717 (-81, -26) -> (-79, -26)
  line L718 (-79, -26) -> (-79, -28)
  line L719 (-79, -28) -> (-81, -28)
  line L720 (-81, -28) -> (-81, -26)
  line L721 (-77, -26) -> (-75, -26)
  line L722 (-75, -26) -> (-75, -28)
  line L723 (-75, -28) -> (-77, -28)
  line L724 (-77, -28) -> (-77, -26)
  line L725 (-73, -26) -> (-71, -26)
  line L726 (-71, -26) -> (-71, -28)
  line L727 (-71, -28) -> (-73, -28)
  line L728 (-73, -28) -> (-73, -26)
  line L729 (-69, -26) -> (-67, -26)
  line L730 (-67, -26) -> (-67, -28)
  line L731 (-67, -28) -> (-69, -28)
  line L732 (-69, -28) -> (-69, -26)
  line L733 (-65, -26) -> (-63, -26)
  line L734 (-63, -26) -> (-63, -28)
  line L735 (-63, -28) -> (-65, -28)
  line L736 (-65, -28) -> (-65, -26)
  line L737 (-61, -26) -> (-59, -26)
  line L738 (-59, -26) -> (-59, -28)
  line L739 (-59, -28) -> (-61, -28)
  line L740 (-61, -28) -> (-61, -26)
  line L741 (-57, -26) -> (-55, -26)
  line L742 (-55, -26) -> (-55, -28)
  line L743 (-55, -28) -> (-57, -28)
  line L744 (-57, -28) -> (-57, -26)
  line L745 (-53, -26) -> (-51, -26)
  line L746 (-51, -26) -> (-51, -28)
  line L747 (-51, -28) -> (-53, -28)
  line L748 (-53, -28) -> (-53, -26)
  line L749 (-49, -26) -> (-47, -26)
  line L750 (-47, -26) -> (-47, -28)
  line L751 (-47, -28) -> (-49, -28)
  line L752 (-49, -28) -> (-49, -26)
  line L753 (-45, -26) -> (-43, -26)
  line L754 (-43, -26) -> (-43, -28)
  line L755 (-43, -28) -> (-45, -28)
  line L756 (-45, -28) -> (-45, -26)
  line L757 (-41, -26) -> (-39, -26)
  line L758 (-39, -26) -> (-39, -28)
  line L759 (-39, -28) -> (-41, -28)
  line L760 (-41, -28) -> (-41, -26)
  line L761 (-37, -26) -> (-35, -26)
  line L762 (-35, -26) -> (-35, -28)
  line L763 (-35, -28) -> (-37, -28)
  line L764 (-37, -28) -> (-37, -26)
  line L765 (-33, -26) -> (-31, -26)
  line L766 (-31, -26) -> (-31, -28)
  line L767 (-31, -28) -> (-33, -28)
  line L768 (-33, -28) -> (-33, -26)
  line L769 (-125, -29) -> (-123, -29)
  line L770 (-123, -29) -> (-123, -31)
  line L771 (-123, -31) -> (-125, -31)
  line L772 (-125, -31) -> (-125, -29)
  line L773 (-121, -29) -> (-119, -29)
  line L774 (-119, -29) -> (-119, -31)
  line L775 (-119, -31) -> (-121, -31)
  line L776 (-121, -31) -> (-121, -29)
  line L777 (-117, -29) -> (-115, -29)
  line L778 (-115, -29) -> (-115, -31)
  line L779 (-115, -31) -> (-117, -31)
  line L780 (-117, -31) -> (-117, -29)
  line L781 (-113, -29) -> (-111, -29)
  line L782 (-111, -29) -> (-111, -31)
  line L783 (-111, -31) -> (-113, -31)
  line L784 (-113, -31) -> (-113, -29)
  line L785 (-109, -29) -> (-107, -29)
  line L786 (-107, -29) -> (-107, -31)
  line L787 (-107, -31) -> (-109, -31)
  line L788 (-109, -31) -> (-109, -29)
  line L789 (-105, -29) -> (-103, -29)
  line L790 (-103, -29) -> (-103, -31)
  line L791 (-103, -31) -> (-105, -31)
  line L792 (-105, -31) -> (-105, -29)
  line L793 (-101, -29) -> (-99, -29)
  line L794 (-99, -29) -> (-99, -31)
  line L795 (-99, -31) -> (-101, -31)
  line L796 (-101, -31) -> (-101, -29)
  line L797 (-97, -29) -> (-95, -29)
  line L798 (-95, -29) -> (-95, -31)
  line L799 (-95, -31) -> (-97, -31)
  line L800 (-97, -31) -> (-97, -29)
  line L801 (-93, -29) -> (-91, -29)
  line L802 (-91, -29) -> (-91, -31)
  line L803 (-91, -31) -> (-93, -31)
  line L804 (-93, -31) -> (-93, -29)
  line L805 (-89, -29) -> (-87, -29)
  line L806 (-87, -29) -> (-87, -31)
  line L807 (-87, -31) -> (-89, -31)
  line L808 (-89, -31) -> (-89, -29)
  line L809 (-85, -29) -> (-83, -29)
  line L810 (-83, -29) -> (-83, -31)
  line L811 (-83, -31) -> (-85, -31)
  line L812 (-85, -31) -> (-85, -29)
  line L813 (-81, -29) -> (-79, -29)
  line L814 (-79, -29) -> (-79, -31)
  line L815 (-79, -31) -> (-81, -31)
  line L816 (-81, -31) -> (-81, -29)
  line L817 (-77, -29) -> (-75, -29)
  line L818 (-75, -29) -> (-75, -31)
  line L819 (-75, -31) -> (-77, -31)
  line L820 (-77, -31) -> (-77, -29)
  line L821 (-73, -29) -> (-71, -29)
  line L822 (-71, -29) -> (-71, -31)
  line L823 (-71, -31) -> (-73, -31)
  line L824 (-73, -31) -> (-73, -29)
  line L825 (-69, -29) -> (-67, -29)
  line L826 (-67, -29) -> (-67, -31)
  line L827 (-67, -31) -> (-69, -31)
  line L828 (-69, -31) -> (-69, -29)
  line L829 (-65, -29) -> (-63, -29)
  line L830 (-63, -29) -> (-63, -31)
  line L831 (-63, -31) -> (-65, -31)
  line L832 (-65, -31) -> (-65, -29)
  line L833 (-61, -29) -> (-59, -29)
  line L834 (-59, -29) -> (-59, -31)
  line L835 (-59, -31) -> (-61, -31)
  line L836 (-61, -31) -> (-61, -29)
  line L837 (-57, -29) -> (-55, -29)
  line L838 (-55, -29) -> (-55, -31)
  line L839 (-55, -31) -> (-57, -31)
  line L840 (-57, -31) -> (-57, -29)
  line L841 (-53, -29) -> (-51, -29)
  line L842 (-51, -29) -> (-51, -31)
  line L843 (-51, -31) -> (-53, -31)
  line L844 (-53, -31) -> (-53, -29)
  line L845 (-49, -29) -> (-47, -29)
  line L846 (-47, -29) -> (-47, -31)
  line L847 (-47, -31) -> (-49, -31)
  line L848 (-49, -31) -> (-49, -29)
  line L849 (-45, -29) -> (-43, -29)
  line L850 (-43, -29) -> (-43, -31)
  line L851 (-43, -31) -> (-45, -31)
  line L852 (-45, -31) -> (-45, -29)
  line L853 (-41, -29) -> (-39, -29)
  line L854 (-39, -29) -> (-39, -31)
  line L855 (-39, -31) -> (-41, -31)
  line L856 (-41, -31) -> (-41, -29)
  line L857 (-37, -29) -> (-35, -29)
  line L858 (-35, -29) -> (-35, -31)
  line L859 (-35, -31) -> (-37, -31)
  line L860 (-37, -31) -> (-37, -29)
  line L861 (-33, -29) -> (-31, -29)
  line L862 (-31, -29) -> (-31, -31)
  line L863 (-31, -31) -> (-33, -31)
  line L864 (-33, -31) -> (-33, -29)
  line L865 (-125, -32) -> (-123, -32)
  line L866 (-123, -32) -> (-123, -34)
  line L867 (-123, -34) -> (-125, -34)
  line L868 (-125, -34) -> (-125, -32)
  line L869 (-121, -32) -> (-119, -32)
  line L870 (-119, -32) -> (-119, -34)
  line L871 (-119, -34) -> (-121, -34)
  line L872 (-121, -34) -> (-121, -32)
  line L873 (-117, -32) -> (-115, -32)
  line L874 (-115, -32) -> (-115, -34)
  line L875 (-115, -34) -> (-117, -34)
  line L876 (-117, -34) -> (-117, -32)
  line L877 (-113, -32) -> (-111, -32)
  line L878 (-111, -32) -> (-111, -34)
  line L879 (-111, -34) -> (-113, -34)
  line L880 (-113, -34) -> (-113, -32)
  line L881 (-109, -32) -> (-107, -32)
  line L882 (-107, -32) -> (-107, -34)
  line L883 (-107, -34) -> (-109, -34)
  line L884 (-109, -34) -> (-109, -32)
  line L885 (-105, -32) -> (-103, -32)
  line L886 (-103, -32) -> (-103, -34)
  line L887 (-103, -34) -> (-105, -34)
  line L888 (-105, -34) -> (-105, -32)
  line L889 (-101, -32) -> (-99, -32)
  line L890 (-99, -32) -> (-99, -34)
  line L891 (-99, -34) -> (-101, -34)
  line L892 (-101, -34) -> (-101, -32)
  line L893 (-97, -32) -> (-95, -32)
  line L894 (-95, -32) -> (-95, -34)
  line L895 (-95, -34) -> (-97, -34)
  line L896 (-97, -34) -> (-97, -32)
  line L897 (-93, -32) -> (-91, -32)
  line L898 (-91, -32) -> (-91, -34)
  line L899 (-91, -34) -> (-93, -34)
  line L900 (-93, -34) -> (-93, -32)
  line L901 (-89, -32) -> (-87, -32)
  line L902 (-87, -32) -> (-87, -34)
  line L903 (-87, -34) -> (-89, -34)
  line L904 (-89, -34) -> (-89, -32)
  line L905 (-85, -32) -> (-83, -32)
  line L906 (-83, -32) -> (-83, -34)
  line L907 (-83, -34) -> (-85, -34)
  line L908 (-85, -34) -> (-85, -32)
  line L909 (-81, -32) -> (-79, -32)
  line L910 (-79, -32) -> (-79, -34)
  line L911 (-79, -34) -> (-81, -34)
  line L912 (-81, -34) -> (-81, -32)
  line L913 (-77, -32) -> (-75, -32)
  line L914 (-75, -32) -> (-75, -34)
  line L915 (-75, -34) -> (-77, -34)
  line L916 (-77, -34) -> (-77, -32)
  line L917 (-73, -32) -> (-71, -32)
  line L918 (-71, -32) -> (-71, -34)
  line L919 (-71, -34) -> (-73, -34)
  line L920 (-73, -34) -> (-73, -32)
  line L921 (-69, -32) -> (-67, -32)
  line L922 (-67, -32) -> (-67, -34)
  line L923 (-67, -34) -> (-69, -34)
  line L924 (-69, -34) -> (-69, -32)
  line L925 (-65, -32) -> (-63, -32)
  line L926 (-63, -32) -> (-63, -34)
  line L927 (-63, -34) -> (-65, -34)
  line L928 (-65, -34) -> (-65, -32)
  line L929 (-61, -32) -> (-59, -32)
  line L930 (-59, -32) -> (-59, -34)
  line L931 (-59, -34) -> (-61, -34)
  line L932 (-61, -34) -> (-61, -32)
  line L933 (-57, -32) -> (-55, -32)
  line L934 (-55, -32) -> (-55, -34)
  line L935 (-55, -34) -> (-57, -34)
  line L936 (-57, -34) -> (-57, -32)
  line L937 (-53, -32) -> (-51, -32)
  line L938 (-51, -32) -> (-51, -34)
  line L939 (-51, -34) -> (-53, -34)
  line L940 (-53, -34) -> (-53, -32)
  line L941 (-49, -32) -> (-47, -32)
  line L942 (-47, -32) -> (-47, -34)
  line L943 (-47, -34) -> (-49, -34)
  line L944 (-49, -34) -> (-49, -32)
  line L945 (-45, -32) -> (-43, -32)
  line L946 (-43, -32) -> (-43, -34)
  line L947 (-43, -34) -> (-45, -34)
  line L948 (-45, -34) -> (-45, -32)
  line L949 (-41, -32) -> (-39, -32)
  line L950 (-39, -32) -> (-39, -34)
  line L951 (-39, -34) -> (-41, -34)
  line L952 (-41, -34) -> (-41, -32)
  line L953 (-37, -32) -> (-35, -32)
  line L954 (-35, -32) -> (-35, -34)
  line L955 (-35, -34) -> (-37, -34)
  line L956 (-37, -34) -> (-37, -32)
  line L957 (-33, -32) -> (-31, -32)
  line L958 (-31, -32) -> (-31, -34)
  line L959 (-31, -34) -> (-33, -34)
  line L960 (-33, -34) -> (-33, -32)
  line L961 (-125, -35) -> (-123, -35)
  line L962 (-123, -35) -> (-123, -37)
  line L963 (-123, -37) -> (-125, -37)
  line L964 (-125, -37) -> (-125, -35)
  line L965 (-121, -35) -> (-119, -35)
  line L966 (-119, -35) -> (-119, -37)
  line L967 (-119, -37) -> (-121, -37)
  line L968 (-121, -37) -> (-121, -35)
  line L969 (-117, -35) -> (-115, -35)
  line L970 (-115, -35) -> (-115, -37)
  line L971 (-115, -37) -> (-117, -37)
  line L972 (-117, -37) -> (-117, -35)
  line L973 (-113, -35) -> (-111, -35)
  line L974 (-111, -35) -> (-111, -37)
  line L975 (-111, -37) -> (-113, -37)
  line L976 (-113, -37) -> (-113, -35)
  line L977 (-109, -35) -> (-107, -35)
  line L978 (-107, -35) -> (-107, -37)
  line L979 (-107, -37) -> (-109, -37)
  line L980 (-109, -37) -> (-109, -35)
  line L981 (-105, -35) -> (-103, -35)
  line L982 (-103, -35) -> (-103, -37)
  line L983 (-103, -37) -> (-105, -37)
  line L984 (-105, -37) -> (-105, -35)
  line L985 (-101, -35) -> (-99, -35)
  line L986 (-99, -35) -> (-99, -37)
  line L987 (-99, -37) -> (-101, -37)
  line L988 (-101, -37) -> (-101, -35)
  line L989 (-97, -35) -> (-95, -35)
  line L990 (-95, -35) -> (-95, -37)
  line L991 (-95, -37) -> (-97, -37)
  line L992 (-97, -37) -> (-97, -35)
  line L993 (-93, -35) -> (-91, -35)
  line L994 (-91, -35) -> (-91, -37)
  line L995 (-91, -37) -> (-93, -37)
  line L996 (-93, -37) -> (-93, -35)
  line L997 (-89, -35) -> (-87, -35)
  line L998 (-87, -35) -> (-87, -37)
  line L999 (-87, -37) -> (-89, -37)
  line L1000 (-89, -37) -> (-89, -35)
  line L1001 (-85, -35) -> (-83, -35)
  line L1002 (-83, -35) -> (-83, -37)
  line L1003 (-83, -37) -> (-85, -37)
  line L1004 (-85, -37) -> (-85, -35)
  line L1005 (-81, -35) -> (-79, -35)
  line L1006 (-79, -35) -> (-79, -37)
  line L1007 (-79, -37) -> (-81, -37)
  line L1008 (-81, -37) -> (-81, -35)
  line L1009 (-77, -35) -> (-75, -35)
  line L1010 (-75, -35) -> (-75, -37)
  line L1011 (-75, -37) -> (-77, -37)
  line L1012 (-77, -37) -> (-77, -35)
  line L1013 (-73, -35) -> (-71, -35)
  line L1014 (-71, -35) -> (-71, -37)
  line L1015 (-71, -37) -> (-73, -37)
  line L1016 (-73, -37) -> (-73, -35)
  line L1017 (-69, -35) -> (-67, -35)
  line L1018 (-67, -35) -> (-67, -37)
  line L1019 (-67, -37) -> (-69, -37)
  line L1020 (-69, -37) -> (-69, -35)
  line L1021 (-65, -35) -> (-63, -35)
  line L1022 (-63, -35) -> (-63, -37)
  line L1023 (-63, -37) -> (-65, -37)
  line L1024 (-65, -37) -> (-65, -35)
  line L1025 (-61, -35) -> (-59, -35)
  line L1026 (-59, -35) -> (-59, -37)
  line L1027 (-59, -37) -> (-61, -37)
  line L1028 (-61, -37) -> (-61, -35)
  line L1029 (-57, -35) -> (-55, -35)
  line L1030 (-55, -35) -> (-55, -37)
  line L1031 (-55, -37) -> (-57, -37)
  line L1032 (-57, -37) -> (-57, -35)
  line L1033 (-53, -35) -> (-51, -35)
  line L1034 (-51, -35) -> (-51, -37)
  line L1035 (-51, -37) -> (-53, -37)
  line L1036 (-53, -37) -> (-53, -35)
  line L1037 (-49, -35) -> (-47, -35)
  line L1038 (-47, -35) -> (-47, -37)
  line L1039 (-47, -37) -> (-49, -37)
  line L1040 (-49, -37) -> (-49, -35)
  line L1041 (-45, -35) -> (-43, -35)
  line L1042 (-43, -35) -> (-43, -37)
  line L1043 (-43, -37) -> (-45, -37)
  line L1044 (-45, -37) -> (-45, -35)
  line L1045 (-41, -35) -> (-39, -35)
  line L1046 (-39, -35) -> (-39, -37)
  line L1047 (-39, -37) -> (-41, -37)
  line L1048 (-41, -37) -> (-41, -35)
  line L1049 (-37, -35) -> (-35, -35)
  line L1050 (-35, -35) -> (-35, -37)
  line L1051 (-35, -37) -> (-37, -37)
  line L1052 (-37, -37) -> (-37, -35)
  line L1053 (-33, -35) -> (-31, -35)
  line L1054 (-31, -35) -> (-31, -37)
  line L1055 (-31, -37) -> (-33, -37)
  line L1056 (-33, -37) -> (-33, -35)
  line L1057 (-125, -38) -> (-123, -38)
  line L1058 (-123, -38) -> (-123, -40)
  line L1059 (-123, -40) -> (-125, -40)
  line L1060 (-125, -40) -> (-125, -38)
  line L1061 (-121, -38) -> (-119, -38)
  line L1062 (-119, -38) -> (-119, -40)
  line L1063 (-119, -40) -> (-121, -40)
  line L1064 (-121, -40) -> (-121, -38)
  line L1065 (-117, -38) -> (-115, -38)
  line L1066 (-115, -38) -> (-115, -40)
  line L1067 (-115, -40) -> (-117, -40)
  line L1068 (-117, -40) -> (-117, -38)
  line L1069 (-113, -38) -> (-111, -38)
  line L1070 (-111, -38) -> (-111, -40)
  line L1071 (-111, -40) -> (-113, -40)
  line L1072 (-113, -40) -> (-113, -38)
  line L1073 (-109, -38) -> (-107, -38)
  line L1074 (-107, -38) -> (-107, -40)
  line L1075 (-107, -40) -> (-109, -40)
  line L1076 (-109, -40) -> (-109, -38)
  line L1077 (-105, -38) -> (-103, -38)
  line L1078 (-103, -38) -> (-103, -40)
  line L1079 (-103, -40) -> (-105, -40)
  line L1080 (-105, -40) -> (-105, -38)
  line L1081 (-101, -38) -> (-99, -38)
  line L1082 (-99, -38) -> (-99, -40)
  line L1083 (-99, -40) -> (-101, -40)
  line L1084 (-101, -40) -> (-101, -38)
  line L1085 (-97, -38) -> (-95, -38)
  line L1086 (-95, -38) -> (-95, -40)
  line L1087 (-95, -40) -> (-97, -40)
  line L1088 (-97, -40) -> (-97, -38)
  line L1089 (-93, -38) -> (-91, -38)
  line L1090 (-91, -38) -> (-91, -40)
  line L1091 (-91, -40) -> (-93, -40)
  line L1092 (-93, -40) -> (-93, -38)
  line L1093 (-89, -38) -> (-87, -38)
  line L1094 (-87, -38) -> (-87, -40)
  line L1095 (-87, -40) -> (-89, -40)
  line L1096 (-89, -40) -> (-89, -38)
  line L1097 (-85, -38) -> (-83, -38)
  line L1098 (-83, -38) -> (-83, -40)
  line L1099 (-83, -40) -> (-85, -40)
  line L1100 (-85, -40) -> (-85, -38)
  line L1101 (-81, -38) -> (-79, -38)
  line L1102 (-79, -38) -> (-79, -40)
  line L1103 (-79, -40) -> (-81, -40)
  line L1104 (-81, -40) -> (-81, -38)
  line L1105 (-77, -38) -> (-75, -38)
  line L1106 (-75, -38) -> (-75, -40)
  line L1107 (-75, -40) -> (-77, -40)
  line L1108 (-77, -40) -> (-77, -38)
  line L1109 (-73, -38) -> (-71, -38)
  line L1110 (-71, -38) -> (-71, -40)
  line L1111 (-71, -40) -> (-73, -40)
  line L1112 (-73, -40) -> (-73, -38)
  line L1113 (-69, -38) -> (-67, -38)
  line L1114 (-67, -38) -> (-67, -40)
  line L1115 (-67, -40) -> (-69, -40)
  line L1116 (-69, -40) -> (-69, -38)
  line L1117 (-65, -38) -> (-63, -38)
  line L1118 (-63, -38) -> (-63, -40)
  line L1119 (-63, -40) -> (-65, -40)
  line L1120 (-65, -40) -> (-65, -38)
  line L1121 (-61, -38) -> (-59, -38)
  line L1122 (-59, -38) -> (-59, -40)
  line L1123 (-59, -40) -> (-61, -40)
  line L1124 (-61, -40) -> (-61, -38)
  line L1125 (-57, -38) -> (-55, -38)
  line L1126 (-55, -38) -> (-55, -40)
  line L1127 (-55, -40) -> (-57, -40)
  line L1128 (-57, -40) -> (-57, -38)
  line L1129 (-53, -38) -> (-51, -38)
  line L1130 (-51, -38) -> (-51, -40)
  line L1131 (-51, -40) -> (-53, -40)
  line L1132 (-53, -40) -> (-53, -38)
  line L1133 (-49, -38) -> (-47, -38)
  line L1134 (-47, -38) -> (-47, -40)
  line L1135 (-47, -40) -> (-49, -40)
  line L1136 (-49, -40) -> (-49, -38)
  line L1137 (-45, -38) -> (-43, -38)
  line L1138 (-43, -38) -> (-43, -40)
  line L1139 (-43, -40) -> (-45, -40)
  line L1140 (-45, -40) -> (-45, -38)
  line L1141 (-41, -38) -> (-39, -38)
  line L1142 (-39, -38) -> (-39, -40)
  line L1143 (-39, -40) -> (-41, -40)
  line L1144 (-41, -40) -> (-41, -38)
  line L1145 (-37, -38) -> (-35, -38)
  line L1146 (-35, -38) -> (-35, -40)
  line L1147 (-35, -40) -> (-37, -40)
  line L1148 (-37, -40) -> (-37, -38)
  line L1149 (-33, -38) -> (-31, -38)
  line L1150 (-31, -38) -> (-31, -40)
  line L1151 (-31, -40) -> (-33, -40)
  line L1152 (-33, -40) -> (-33, -38)
  point P0 (0, 0)
  point P1 (-124, -5)
  point P2 (-128, -22.5)
  point P3 (-125, -6)
  point P4 (-120, -5)
  point P5 (-121, -6)
  point P6 (-116, -5)
  point P7 (-117, -6)
  point P8 (-112, -5)
  point P9 (-113, -6)
  point P10 (-108, -5)
  point P11 (-109, -6)
  point P12 (-104, -5)
  point P13 (-105, -6)
  point P14 (-100, -5)
  point P15 (-101, -6)
  point P16 (-96, -5)
  point P17 (-97, -6)
  point P18 (-92, -5)
  point P19 (-93, -6)
  point P20 (-88, -5)
  point P21 (-89, -6)
  point P22 (-84, -5)
  point P23 (-85, -6)
  point P24 (-80, -5)
  point P25 (-81, -6)
  point P26 (-76, -5)
  point P27 (-77, -6)
  point P28 (-72, -5)
  point P29 (-73, -6)
  point P30 (-68, -5)
  point P31 (-69, -6)
  point P32 (-64, -5)
  point P33 (-65, -6)
  point P34 (-60, -5)
  point P35 (-61, -6)
  point P36 (-56, -5)
  point P37 (-57, -6)
  point P38 (-52, -5)
  point P39 (-53, -6)
  point P40 (-48, -5)
  point P41 (-49, -6)
  point P42 (-44, -5)
  point P43 (-45, -6)
  point P44 (-40, -5)
  point P45 (-41, -6)
  point P46 (-36, -5)
  point P47 (-37, -6)
  point P48 (-32, -5)
  point P49 (-33, -6)
  point P50 (-124, -8)
  point P51 (-125, -9)
  point P52 (-120, -8)
  point P53 (-121, -9)
  point P54 (-116, -8)
  point P55 (-117, -9)
  point P56 (-112, -8)
  point P57 (-113, -9)
  point P58 (-108, -8)
  point P59 (-109, -9)
  point P60 (-104, -8)
  point P61 (-105, -9)
  point P62 (-100, -8)
  point P63 (-101, -9)
  point P64 (-96, -8)
  point P65 (-97, -9)
  point P66 (-92, -8)
  point P67 (-93, -9)
  point P68 (-88, -8)
  point P69 (-89, -9)
  point P70 (-84, -8)
  point P71 (-85, -9)
  point P72 (-80, -8)
  point P73 (-81, -9)
  point P74 (-76, -8)
  point P75 (-77, -9)
  point P76 (-72, -8)
  point P77 (-73, -9)
  point P78 (-68, -8)
  point P79 (-69, -9)
  point P80 (-64, -8)
  point P81 (-65, -9)
  point P82 (-60, -8)
  point P83 (-61, -9)
  point P84 (-56, -8)
  point P85 (-57, -9)
  point P86 (-52, -8)
  point P87 (-53, -9)
  point P88 (-48, -8)
  point P89 (-49, -9)
  point P90 (-44, -8)
  point P91 (-45, -9)
  point P92 (-40, -8)
  point P93 (-41, -9)
  point P94 (-36, -8)
  point P95 (-37, -9)
  point P96 (-32, -8)
  point P97 (-33, -9)
  point P98 (-124, -11)
  point P99 (-125, -12)
  point P100 (-120, -11)
  point P101 (-121, -12)
  point P102 (-116, -11)
  point P103 (-117, -12)
  point P104 (-112, -11)
  point P105 (-113, -12)
  point P106 (-108, -11)
  point P107 (-109, -12)
  point P108 (-104, -11)
  point P109 (-105, -12)
  point P110 (-100, -11)
  point P111 (-101, -12)
  point P112 (-96, -11)
  point P113 (-97, -12)
  point P114 (-92, -11)
  point P115 (-93, -12)
  point P116 (-88, -11)
  point P117 (-89, -12)
  point P118 (-84, -11)
  point P119 (-85, -12)
  point P120 (-80, -11)
  point P121 (-81, -12)
  point P122 (-76, -11)
  point P123 (-77, -12)
  point P124 (-72, -11)
  point P125 (-73, -12)
  point P126 (-68, -11)
  point P127 (-69, -12)
  point P128 (-64, -11)
  point P129 (-65, -12)
  point P130 (-60, -11)
  point P131 (-61, -12)
  point P132 (-56, -11)
  point P133 (-57, -12)
  point P134 (-52, -11)
  point P135 (-53, -12)
  point P136 (-48, -11)
  point P137 (-49, -12)
  point P138 (-44, -11)
  point P139 (-45, -12)
  point P140 (-40, -11)
  point P141 (-41, -12)
  point P142 (-36, -11)
  point P143 (-37, -12)
  point P144 (-32, -11)
  point P145 (-33, -12)
  point P146 (-124, -14)
  point P147 (-125, -15)
  point P148 (-120, -14)